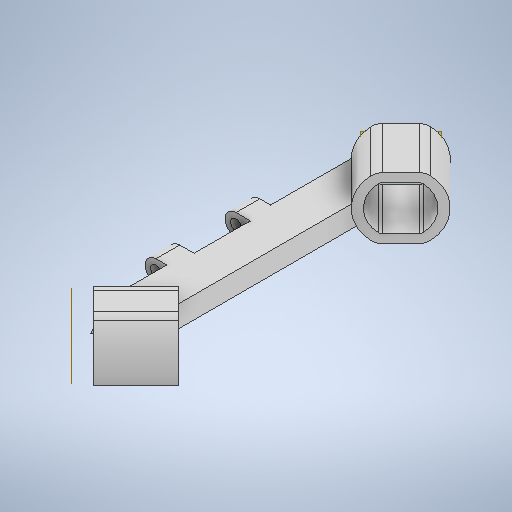
# Autodesk Inventor part: Drib_v1
Saved by Autodesk Inventor 2025.1 (Build 291241000, 241)
## iProperties
Created: 2026-05-05
Part Number: Drib_v1
Material: Generic
Document SubType Name: Modeling
Designer: User
Density: 1 g/cm^3
Appearance: Default
Author: User
## iProperties of the stored document Drib_v1_3DPrint.ipt
Created: 2026-05-05
Part Number: Drib_v1_3DPrint
Material: Generic
Document SubType Name: Modeling
Designer: User
Density: 1 g/cm^3
Appearance: Default
Author: User
Autodesk Inventor part; units mm, degrees
ref_plane "YZ Plane" through (0, 0, 0) normal (1, 0, 0) x (0, 1, 0)
ref_plane "XZ Plane" through (0, 0, 0) normal (0, 1, 0) x (-1, 0, 0)
ref_plane "XY Plane" through (0, 0, 0) normal (0, 0, 1) x (1, 0, 0)
sketch "Sketch1" plane through (0, 0, 0) normal (0, 0, 1) x (1, 0, 0)
  circle A0 centre (-3, -3.25) radius 1.25 projected
  line L0 (-6, -6.5) -> (-6, 0) projected
  circle A1 centre (-3, -3.25) radius 2.5
  point P0 (0, 0)
  dimension "d0" = 5
  constraints: 1 centre point, 1 coincident
  measures "d0" diameter of A1
extrude "Extrusion1" add sketch "Sketch1" along normal blind 6
sketch "Sketch2" plane through (-3, -3.25, 6) normal (0, 0, 1) x (1, 0, 0)
  arc A0 (3, 0.25) -> (0, 3.25) centre (0, 0.25) ccw projected
  line L0 (3, 0.25) -> (3, -0.25) projected
  arc A1 (0, -3.25) -> (3, -0.25) centre (0, -0.25) ccw projected
  arc A2 (4, 0.25) -> (0, 4.25) centre (0, 0.25) ccw
  line L1 (4, 0.25) -> (4, -0.25)
  arc A3 (0, -4.25) -> (4, -0.25) centre (0, -0.25) ccw
  circle A4 centre (0, 0) radius 2.5 projected
  circle A5 centre (0, 0) radius 2.5 projected
  line L2 (0, -2.5) -> (3.3072, -2.5)
  arc A6 (7, 0.25) -> (0, 7.25) centre (0, 0.25) ccw
  line L3 (7, 0.25) -> (7, -0.25)
  arc A7 (0, -7.25) -> (7, -0.25) centre (0, -0.25) ccw
  line L4 (0, 2.5) -> (6.6285, 2.5)
  line L5 (0, 2.5) -> (6.6285, 2.5) construction
  line L6 (0, -2.5) -> (6.6285, -2.5)
  line L7 (0, -2.5) -> (6.6285, -2.5) construction
  point P0 (3, 3.25)
  point P1 (3.3072, -2.5)
  point P2 (0, -2.5)
  dimension "d0" = 5
  dimension "d3" = 1
  dimension "d4" = 3
  dimension "d5" = 0
  dimension "d6" = 0
  constraints: 14 end point, 13 point on circle, 4 centre point, 3 horizontal, 2 collinear, 2 tangent, 4 other
  measures "d3" radial gap between concentric circles of A0 A2
  measures "d4" radial gap between concentric circles of A2 A6
  measures "d5" distance between parallel lines of L4 L5
  measures "d6" distance between parallel lines of L7 L6
extrude "Extrusion2" add sketch "Sketch2" against normal blind 6 contours L0 A1 L2 A4 L4 A0 | A0 L4 A2 L1 A3 L2 A1 L0 | L4 A6 L3 A7 L6 A3 L1 A2
sketch "Sketch3" plane through (0, 0, 0) normal (0, 0, -1) x (-1, 0, 0)
  line L0 (3, -0.75) -> (-3.6285, -0.75) projected
  arc A0 (-3.6285, -0.75) -> (-4, -3) centre (3, -3) ccw projected
  line L1 (-4, -3) -> (-4, -3.5) projected
  arc A1 (-4, -3.5) -> (-3.6285, -5.75) centre (3, -3.5) ccw projected
  line L2 (-3.6285, -5.75) -> (3, -5.75) projected
  arc A2 (3, -5.75) -> (3, -0.75) centre (3, -3.25) ccw projected
  circle A3 centre (3, -3.25) radius 1.25 projected
  point P0 (0, 0)
extrude "Extrusion3" cut sketch "Sketch3" against normal blind 0.5
sketch "Sketch4" plane through (0, 0, 0.5) normal (0, 0, -1) x (-1, 0, 0)
  arc A0 (3, 0) -> (0, -3) centre (3, -3) ccw projected
  line L0 (0, -3) -> (0, -3.5) projected
  arc A1 (0, -3.5) -> (3, -6.5) centre (3, -3.5) ccw projected
  arc A2 (-1, -3.5) -> (3, -7.5) centre (3, -3.5) ccw
  line L1 (-1, -3.5) -> (-1, -3)
  arc A3 (3, 1) -> (-1, -3) centre (3, -3) ccw
  line L2 (-3.6285, -0.75) -> (3, -0.75) projected
  arc A4 (-3.6285, -0.75) -> (-4, -3) centre (3, -3) ccw projected
  line L3 (-4, -3.5) -> (-4, -3) projected
  arc A5 (-4, -3.5) -> (-3.6285, -5.75) centre (3, -3.5) ccw projected
  line L4 (3, -5.75) -> (-3.6285, -5.75) projected
  point P0 (0, 0)
  point P1 (-0.3072, -0.75)
  point P2 (-0.3072, -5.75)
  dimension "d11" = 1
  constraints: 4 point on circle, 2 centre point, 2 end point, 2 other
  measures "d11" distance between parallel lines of L0 L1
ref_plane "Work Plane1" through (-6, -6.5, -12) normal (0, 0, -1) x (0, 1, 0)
extrude "Extrusion4" add sketch "Sketch4" along normal up to surface (12.5 mm away) contours A3 L1 A2 L4 A5 L3 A4 L2
sketch "Sketch5" plane through (3.6285, -0.75, -12) normal (0, 0, -1) x (-1, 0, 0)
  line L0 (2.6285, -2.25) -> (2.6285, -2.75) projected
  arc A0 (3.3213, 0) -> (2.6285, -2.25) centre (6.6285, -2.25) ccw projected
  line L1 (0, 0) -> (3.3213, 0) projected
  arc A1 (0, 0) -> (-0.3715, -2.25) centre (6.6285, -2.25) ccw projected
  line L2 (-0.3715, -2.75) -> (-0.3715, -2.25) projected
  arc A2 (-0.3715, -2.75) -> (0, -5) centre (6.6285, -2.75) ccw projected
  line L3 (3.3213, -5) -> (0, -5) projected
  arc A3 (2.6285, -2.75) -> (3.3213, -5) centre (6.6285, -2.75) ccw projected
  line L4 (2.6285, -2.25) -> (2.6285, -2.75) projected
  arc A4 (3.3213, 0) -> (2.6285, -2.25) centre (6.6285, -2.25) ccw projected
  line L5 (0, 0) -> (3.3213, 0) projected
  arc A5 (0, 0) -> (-0.3715, -2.25) centre (6.6285, -2.25) ccw projected
  line L6 (-0.3715, -2.75) -> (-0.3715, -2.25) projected
  arc A6 (-0.3715, -2.75) -> (0, -5) centre (6.6285, -2.75) ccw projected
  line L7 (3.3213, -5) -> (0, -5) projected
  arc A7 (2.6285, -2.75) -> (3.3213, -5) centre (6.6285, -2.75) ccw projected
  point P0 (3.6285, 0.75)
extrude "Extrusion5" add sketch "Sketch5" along normal blind 0.5
sketch "Sketch6" plane through (3.6285, -0.75, -12.5) normal (0, 0, -1) x (-1, 0, 0)
  arc A0 (6.6285, -5) -> (6.6285, 0) centre (6.6285, -2.5) ccw projected
  line L0 (6.6285, -5) -> (0, -5) projected
  arc A1 (-0.3715, -2.75) -> (0, -5) centre (6.6285, -2.75) ccw projected
  line L1 (-0.3715, -2.75) -> (-0.3715, -2.25) projected
  arc A2 (0, 0) -> (-0.3715, -2.25) centre (6.6285, -2.25) ccw projected
  line L2 (0, 0) -> (6.6285, 0) projected
  circle A3 centre (6.6285, -2.5) radius 1.25 projected
  point P0 (3.6285, 0.75)
  dimension "d3" = 1
  dimension "d4" = 3
  dimension "d5" = 0
  dimension "d6" = 0
extrude "Extrusion6" add sketch "Sketch6" along normal blind 5.5
ref_plane "Work Plane2" through (-3.2559, 6.1157, 25.3527) normal (-0.7077026, 0, 0.7065105) x (0.7065105, 0, 0.7077026)
sketch "Sketch7" plane through (-3.2559, 6.1157, 25.3527) normal (-0.7077026, 0, 0.7065105) x (0.7065105, 0, 0.7077026)
  arc A0 (11.1, -12.3) -> (11.1, -2.7) centre (7.5, -7.5) ccw projected
  arc A1 (11.1, -2.7) -> (10.5, -2.5) centre (10.5, -3.5) ccw projected
  line L0 (10.5, -2.5) -> (4.5, -2.5) projected
  arc A2 (4.5, -2.5) -> (3.9, -2.7) centre (4.5, -3.5) ccw projected
  arc A3 (3.9, -2.7) -> (3.9, -12.3) centre (7.5, -7.5) ccw projected
  arc A4 (3.9, -12.3) -> (4.5, -12.5) centre (4.5, -11.5) ccw projected
  line L1 (4.5, -12.5) -> (10.5, -12.5) projected
  arc A5 (10.5, -12.5) -> (11.1, -12.3) centre (10.5, -11.5) ccw projected
  arc A6 (3.84, -2.62) -> (3.84, -12.38) centre (7.5, -7.5) ccw
  arc A7 (4.5, -2.4) -> (3.84, -2.62) centre (4.5, -3.5) ccw
  line L2 (4.5, -2.4) -> (10.5, -2.4)
  arc A8 (11.16, -2.62) -> (10.5, -2.4) centre (10.5, -3.5) ccw
  arc A9 (11.16, -12.38) -> (11.16, -2.62) centre (7.5, -7.5) ccw
  arc A10 (10.5, -12.6) -> (11.16, -12.38) centre (10.5, -11.5) ccw
  line L3 (10.5, -12.6) -> (4.5, -12.6)
  arc A11 (3.84, -12.38) -> (4.5, -12.6) centre (4.5, -11.5) ccw
  arc A12 (2.64, -1.02) -> (2.64, -13.98) centre (7.5, -7.5) ccw
  arc A13 (4.5, -0.4) -> (2.64, -1.02) centre (4.5, -3.5) ccw
  line L4 (4.5, -0.4) -> (10.5, -0.4)
  arc A14 (12.36, -1.02) -> (10.5, -0.4) centre (10.5, -3.5) ccw
  arc A15 (12.36, -13.98) -> (12.36, -1.02) centre (7.5, -7.5) ccw
  arc A16 (10.5, -14.6) -> (12.36, -13.98) centre (10.5, -11.5) ccw
  line L5 (10.5, -14.6) -> (4.5, -14.6)
  arc A17 (2.64, -13.98) -> (4.5, -14.6) centre (4.5, -11.5) ccw
  point P0 (-15.6418, -6.1157)
  dimension "d18" = 0.1
  dimension "d19" = 2
  constraints: 24 point on circle, 12 centre point, 8 end point, 14 other
  measures "d18" radial gap between concentric circles of A3 A6
  measures "d19" radial gap between concentric circles of A6 A12
ref_plane "Work Plane3" through (8.5556, -6.2866, 15.8116) normal (-0.7077026, 0, 0.7065105) x (0.7065105, 0, 0.7077026)
extrude "Extrusion7" add sketch "Sketch7" against normal up to surface (15.1 mm away) contours A13 L4 A14 A15 A16 L5 A17 A12
ref_plane "Work Plane4" through (18.8366, 4.7079, -57.0191) normal (-0.7066713, 0, -0.707542) x (-0.707542, 0, 0.7066713)
sketch "Sketch8" plane through (18.8366, 4.7079, -57.0191) normal (-0.7066713, 0, -0.707542) x (-0.707542, 0, 0.7066713)
  line L0 (23, -1.1) -> (17, -1.1) projected
  arc A0 (17, -1.1) -> (16.4, -1.3) centre (17, -2.1) ccw projected
  arc A1 (16.4, -1.3) -> (16.4, -10.9) centre (20, -6.1) ccw projected
  arc A2 (16.4, -10.9) -> (17, -11.1) centre (17, -10.1) ccw projected
  line L1 (17, -11.1) -> (23, -11.1) projected
  arc A3 (23, -11.1) -> (23.6, -10.9) centre (23, -10.1) ccw projected
  arc A4 (23.6, -10.9) -> (23.6, -1.3) centre (20, -6.1) ccw projected
  arc A5 (23.6, -1.3) -> (23, -1.1) centre (23, -2.1) ccw projected
  line L2 (17, -1) -> (23, -1)
  arc A6 (23.66, -1.22) -> (23, -1) centre (23, -2.1) ccw
  arc A7 (23.66, -10.98) -> (23.66, -1.22) centre (20, -6.1) ccw
  arc A8 (23, -11.2) -> (23.66, -10.98) centre (23, -10.1) ccw
  line L3 (23, -11.2) -> (17, -11.2)
  arc A9 (16.34, -10.98) -> (17, -11.2) centre (17, -10.1) ccw
  arc A10 (16.34, -1.22) -> (16.34, -10.98) centre (20, -6.1) ccw
  arc A11 (17, -1) -> (16.34, -1.22) centre (17, -2.1) ccw
  line L4 (23, 1) -> (17, 1)
  arc A12 (17, 1) -> (15.14, 0.38) centre (17, -2.1) ccw
  arc A13 (15.14, 0.38) -> (15.14, -12.58) centre (20, -6.1) ccw
  arc A14 (15.14, -12.58) -> (17, -13.2) centre (17, -10.1) ccw
  line L5 (17, -13.2) -> (23, -13.2)
  arc A15 (23, -13.2) -> (24.86, -12.58) centre (23, -10.1) ccw
  arc A16 (24.86, -12.58) -> (24.86, 0.38) centre (20, -6.1) ccw
  arc A17 (24.86, 0.38) -> (23, 1) centre (23, -2.1) ccw
  point P0 (53.6215, -4.7079)
  dimension "d22" = 0.1
  dimension "d23" = 2
  constraints: 24 point on circle, 12 centre point, 8 end point, 14 other
  measures "d22" distance between parallel lines of L0 L2
  measures "d23" distance between parallel lines of L2 L4
ref_plane "Work Plane5" through (14.5059, -6.2945, -33.0483) normal (-0.7066713, 0, -0.707542) x (0, 1, 0)
extrude "Extrusion8" add sketch "Sketch8" against normal up to surface (13.9 mm away) contours A17 A16 A15 L5 A14 A13 A12 L4
sketch "Sketch9" plane through (0, 0, 6) normal (0, 0, 1) x (1, 0, 0)
  arc A0 (-3, -0.75) -> (-3, -5.75) centre (-3, -3.25) ccw projected
  circle A1 centre (-3, -3.25) radius 2.5
  arc A2 (-3, -0.75) -> (-3, -5.75) centre (-3, -3.25) ccw projected
  line L0 (-3, -5.75) -> (3.6285, -5.75) projected
  arc A3 (3.6285, -5.75) -> (4, -3.5) centre (-3, -3.5) ccw projected
  line L1 (4, -3.5) -> (4, -3) projected
  arc A4 (4, -3) -> (3.6285, -0.75) centre (-3, -3) ccw projected
  line L2 (3.6285, -0.75) -> (-3, -0.75) projected
  circle A5 centre (-3, -3.25) radius 1.25 projected
  line L3 (3.6285, -0.75) -> (-3, -0.75) projected
  line L4 (-0.5, -0.75) -> (-0.5, -5.75)
  point P0 (0, 0)
  constraints: 2 end point, 2 point on line, 1 centre point, 1 coincident, 1 concentric, 1 perpendicular
extrude "Extrusion9" add sketch "Sketch9" along normal up to surface contours L4 L2 A4 L1 A3 L0 round surface about axis through (2.0429, -1.3843, 30.6605) along (0.7077026, 0, -0.7065105) radius 8.1 far side no
sketch "Sketch10" plane through (3.6285, -0.75, -18) normal (0, 0, -1) x (-1, 0, 0)
  line L0 (4.1285, -5) -> (4.1285, 0) projected
  line L1 (0, 0) -> (0, 0) projected
  spline S0 degree 5 poles (-0.3715, -2.25) (-0.3715, -2.2011) (-0.371, -2.1517) (-0.3702, -2.1016) (-0.3688, -2.051) (-0.3635, -1.9016) (-0.3582, -1.8015) (-0.351, -1.7001) (-0.3418, -1.598) (-0.3181, -1.3795) (-0.3031, -1.2634) (-0.2857, -1.1483) (-0.2662, -1.0352) (-0.2329, -0.8626) (-0.2203, -0.8012) (-0.2072, -0.7408) (-0.1937, -0.6812) (-0.1473, -0.4872) (-0.1127, -0.3574) (-0.0764, -0.233) (-0.0387, -0.114) (0, 0) knots 0 0 0 0 0 0 0.108522 0.108522 0.108522 0.108522 0.317166 0.317166 0.317166 0.317166 0.554891 0.554891 0.554891 0.554891 0.689067 0.689067 0.689067 0.689067 1 1 1 1 1 1 projected
  line L2 (-0.3715, -2.25) -> (-0.3715, -2.25) projected
  arc A0 (0, 0) -> (-0.3715, -2.25) centre (6.6285, -2.25) ccw projected
  line L3 (0, -5) -> (6.6285, -5) projected
  arc A1 (6.6285, -5) -> (6.6285, 0) centre (6.6285, -2.5) ccw projected
  line L4 (6.6285, 0) -> (0, 0) projected
  arc A2 (0, 0) -> (-0.3715, -2.25) centre (6.6285, -2.25) ccw projected
  line L5 (-0.3715, -2.25) -> (-0.3715, -2.75) projected
  arc A3 (-0.3715, -2.75) -> (0, -5) centre (6.6285, -2.75) ccw projected
  circle A4 centre (6.6285, -2.5) radius 1.25 projected
  point P0 (3.6285, 0.75)
  point P1 (4.1285, 0)
  point P2 (0, 0)
  point P3 (-0.3715, -2.25)
  dimension "d3" = 1
  dimension "d4" = 3
  dimension "d5" = 0
  dimension "d6" = 0
  constraints: 1 other
extrude "Extrusion10" add sketch "Sketch10" along normal up to surface contours L3 A3 L5 S0 L4 L0 round surface about axis through (4.6858, -1.3921, -42.8857) along (0.7066713, 0, 0.707542) radius 8.1 far side no
sketch "Sketch11" plane through (-3.2559, 6.1157, 25.3527) normal (-0.7077026, 0, 0.7065105) x (0.7065105, 0, 0.7077026)
  arc A0 (2.64, -1.02) -> (2.64, -13.98) centre (7.5, -7.5) ccw projected
  arc A1 (2.64, -13.98) -> (4.5, -14.6) centre (4.5, -11.5) ccw projected
  line L0 (4.5, -14.6) -> (10.5, -14.6) projected
  arc A2 (10.5, -14.6) -> (12.36, -13.98) centre (10.5, -11.5) ccw projected
  arc A3 (12.36, -13.98) -> (12.36, -1.02) centre (7.5, -7.5) ccw projected
  arc A4 (12.36, -1.02) -> (10.5, -0.4) centre (10.5, -3.5) ccw projected
  line L1 (10.5, -0.4) -> (4.5, -0.4) projected
  arc A5 (4.5, -0.4) -> (2.64, -1.02) centre (4.5, -3.5) ccw projected
  line L2 (4.5, -2.4) -> (10.5, -2.4) projected
  arc A6 (11.16, -2.62) -> (10.5, -2.4) centre (10.5, -3.5) ccw projected
  arc A7 (11.16, -12.38) -> (11.16, -2.62) centre (7.5, -7.5) ccw projected
  arc A8 (10.5, -12.6) -> (11.16, -12.38) centre (10.5, -11.5) ccw projected
  line L3 (10.5, -12.6) -> (4.5, -12.6) projected
  arc A9 (3.84, -12.38) -> (4.5, -12.6) centre (4.5, -11.5) ccw projected
  arc A10 (3.84, -2.62) -> (3.84, -12.38) centre (7.5, -7.5) ccw projected
  arc A11 (4.5, -2.4) -> (3.84, -2.62) centre (4.5, -3.5) ccw projected
  point P0 (-15.6418, -6.1157)
ref_plane "Work Plane6" through (-1.3505, -6.3843, 25.5629) normal (0.7077026, 0, -0.7065105) x (0, 1, 0)
extrude "Extrusion11" cut sketch "Sketch11" against normal up to surface (1.2 mm away)
sketch "Sketch12" plane through (0, 0, 0.5) normal (0, 0, -1) x (-1, 0, 0)
  spline S0 degree 5 poles (-4, -3) (-4, -2.9511) (-3.9996, -2.9017) (-3.9987, -2.8516) (-3.9974, -2.801) (-3.992, -2.6516) (-3.9867, -2.5515) (-3.9795, -2.4501) (-3.9703, -2.348) (-3.9467, -2.1295) (-3.9316, -2.0134) (-3.9142, -1.8983) (-3.8947, -1.7852) (-3.8614, -1.6126) (-3.8489, -1.5512) (-3.8358, -1.4908) (-3.8222, -1.4312) (-3.7758, -1.2372) (-3.7412, -1.1074) (-3.7049, -0.983) (-3.6672, -0.864) (-3.6285, -0.75) knots 0 0 0 0 0 0 0.108522 0.108522 0.108522 0.108522 0.317166 0.317166 0.317166 0.317166 0.554891 0.554891 0.554891 0.554891 0.689067 0.689067 0.689067 0.689067 1 1 1 1 1 1 projected
  arc A0 (-3.6285, -0.75) -> (-4, -3) centre (3, -3) ccw projected
  line L0 (-4, -3.5) -> (-4, -3) projected
  line L1 (-4, -3.5) -> (-4, -3) projected
  spline S1 degree 6 poles (-3.6285, -5.75) (-3.6937, -5.558) (-3.7551, -5.3554) (-3.8132, -5.1365) (-3.8673, -4.8961) (-3.9146, -4.6301) (-3.9648, -4.2119) (-3.9776, -4.0831) (-3.9881, -3.948) (-3.9958, -3.8061) (-4, -3.6569) (-4, -3.5) knots 0 0 0 0 0 0 0 0.705577 0.705577 0.705577 0.705577 0.705577 1 1 1 1 1 1 1 projected
  arc A1 (-4, -3.5) -> (-3.6285, -5.75) centre (3, -3.5) ccw projected
  line L2 (-3.6285, -0.75) -> (-8.6285, -0.75)
  line L3 (-3.6285, -5.75) -> (-8.6285, -5.75)
  line L4 (-3.6285, -5.75) -> (1.3715, -5.75) construction
  line L5 (-8.6285, -5.75) -> (-8.6285, -0.75)
  point P0 (0, 0)
  point P1 (-3.6285, -5.75)
  dimension "d32" = 5
  dimension "d33" = 180
  constraints: 8 end point, 2 horizontal, 1 collinear, 1 perpendicular, 2 other
  measures "d32" distance of L2.start L2.end
  measures "d33" angle of L3 L4
extrude "Extrusion12" add sketch "Sketch12" along normal up to surface round surface about axis through (4.6858, -1.3921, -42.8857) along (0.7066713, 0, 0.707542) radius 8.1 far side no
sketch "Sketch13" plane through (0, 0, 0.5) normal (0, 0, 1) x (1, 0, 0)
  line L0 (8.6285, -0.75) -> (8.6285, -5.75) projected
  line L1 (3.6285, -0.75) -> (8.6285, -0.75) projected
  arc A0 (4, -3) -> (3.6285, -0.75) centre (-3, -3) ccw projected
  line L2 (4, -3.5) -> (4, -3) projected
  arc A1 (3.6285, -5.75) -> (4, -3.5) centre (-3, -3.5) ccw projected
  line L3 (8.6285, -5.75) -> (3.6285, -5.75) projected
  point P0 (0, 0)
extrude "Extrusion13" add sketch "Sketch13" along normal up to surface round surface about axis through (2.0429, -1.3843, 30.6605) along (0.7077026, 0, -0.7065105) radius 8.1 far side no
sketch "Sketch14" plane through (0, 0, 6) normal (0, 0, 1) x (1, 0, 0)
  line L0 (-0.5, -5.75) -> (-0.5, -0.75) projected
  line L1 (-0.5, -0.75) -> (-3, -0.75) projected
  arc A0 (-3, -0.75) -> (-3, -5.75) centre (-3, -3.25) ccw projected
  line L2 (-3, -5.75) -> (-0.5, -5.75) projected
  circle A1 centre (-3, -3.25) radius 1.25 projected
  point P0 (0, 0)
extrude "Extrusion14" cut sketch "Sketch14" along normal through all contours L2 A0 L1 L0 | A1
sketch "Sketch15" plane through (12.7292, -1.3843, 19.9922) normal (0.7077026, 0, -0.7065105) x (-0.7065105, 0, -0.7077026)
  arc A0 (-3, 5.1) -> (-3.66, 4.88) centre (-3, 4) ccw projected
  line L0 (-3, 5.1) -> (3, 5.1) projected
  arc A1 (3.66, 4.88) -> (3, 5.1) centre (3, 4) ccw projected
  arc A2 (3.66, -4.88) -> (3.66, 4.88) centre (0, 0) ccw projected
  arc A3 (3, -5.1) -> (3.66, -4.88) centre (3, -4) ccw projected
  line L1 (3, -5.1) -> (-3, -5.1) projected
  arc A4 (-3.66, -4.88) -> (-3, -5.1) centre (-3, -4) ccw projected
  arc A5 (-3.66, 4.88) -> (-3.66, -4.88) centre (0, 0) ccw projected
  arc A6 (3, -7.1) -> (4.86, -6.48) centre (3, -4) ccw projected
  arc A7 (4.86, -6.48) -> (6.8228, -4.3657) centre (0, 0) ccw projected
  arc A8 (6.8228, -4.3657) -> (8.0751, 0.6343) centre (0, 0) ccw projected
  arc A9 (8.0751, 0.6343) -> (4.86, 6.48) centre (0, 0) ccw projected
  arc A10 (4.86, 6.48) -> (3, 7.1) centre (3, 4) ccw projected
  line L2 (3, 7.1) -> (-3, 7.1) projected
  arc A11 (-3, 7.1) -> (-4.86, 6.48) centre (-3, 4) ccw projected
  arc A12 (-4.86, 6.48) -> (-4.86, -6.48) centre (0, 0) ccw projected
  arc A13 (-4.86, -6.48) -> (-3, -7.1) centre (-3, -4) ccw projected
  line L3 (-3, -7.1) -> (3, -7.1) projected
  point P0 (23.1418, 1.3843)
extrude "Extrusion15" add sketch "Sketch15" along normal blind 2.5
sketch "Sketch16" plane through (2.8921, -1.3843, 29.8127) normal (-0.7077026, 0, 0.7065105) x (0.7065105, 0, 0.7077026)
  line L0 (-8.0751, 0.6343) -> (-6.0669, 0.6343) projected
  arc A0 (-3.66, 4.88) -> (-6.0669, 0.6343) centre (0, 0) ccw projected
  arc A1 (-3, 5.1) -> (-3.66, 4.88) centre (-3, 4) ccw projected
  line L1 (3, 5.1) -> (-3, 5.1) projected
  arc A2 (3.66, 4.88) -> (3, 5.1) centre (3, 4) ccw projected
  arc A3 (3.66, -4.88) -> (3.66, 4.88) centre (0, 0) ccw projected
  arc A4 (3, -5.1) -> (3.66, -4.88) centre (3, -4) ccw projected
  line L2 (-3, -5.1) -> (3, -5.1) projected
  arc A5 (-3.66, -4.88) -> (-3, -5.1) centre (-3, -4) ccw projected
  arc A6 (-4.8013, -3.7627) -> (-3.66, -4.88) centre (0, 0) ccw projected
  line L3 (-4.8013, -3.7627) -> (-4.8013, -4.3657) projected
  line L4 (-4.8013, -4.3657) -> (-6.8228, -4.3657) projected
  arc A7 (-6.8228, -4.3657) -> (-4.86, -6.48) centre (0, 0) ccw projected
  arc A8 (-4.86, -6.48) -> (-3, -7.1) centre (-3, -4) ccw projected
  line L5 (3, -7.1) -> (-3, -7.1) projected
  arc A9 (3, -7.1) -> (4.86, -6.48) centre (3, -4) ccw projected
  arc A10 (4.86, -6.48) -> (4.86, 6.48) centre (0, 0) ccw projected
  arc A11 (4.86, 6.48) -> (3, 7.1) centre (3, 4) ccw projected
  line L6 (-3, 7.1) -> (3, 7.1) projected
  arc A12 (-3, 7.1) -> (-4.86, 6.48) centre (-3, 4) ccw projected
  arc A13 (-4.86, 6.48) -> (-8.0751, 0.6343) centre (0, 0) ccw projected
  arc A14 (-6.0669, 0.6343) -> (-4.8013, -3.7627) centre (0, 0) ccw projected
  arc A15 (-8.0561, 0.8423) -> (-6.3754, -4.9964) centre (0, 0) ccw
  point P0 (-23.1418, 1.3843)
  dimension "d42" = 2
  constraints: 2 point on circle, 1 centre point
  measures "d42" radial gap between concentric circles of A14 A15
extrude "Extrusion16" cut sketch "Sketch16" against normal blind 2.5 contours A13 A12 L6 A11 A10 A9 L5 A8 A7 L4 L3 A6 A5 L2 A4 A3 A2 L1 A1 A0 L0 | L0 A14 L3 L4 A15
body "Solid1"
